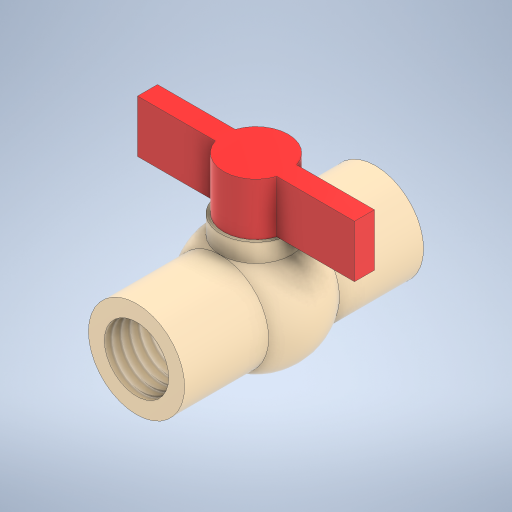
# Autodesk Inventor part: LlaveDesecho
Saved by Autodesk Inventor 2024 (Build 280153000, 153)
## iProperties
Created: 2024-05-01
Part Number: LlaveDesecho
Material: Genérico
Document SubType Name: Modeling
Designer: alexa
Density: 1 g/cm^3
Appearance: Valor por defecto
Author: alexa
Autodesk Inventor part; units mm, degrees
ref_plane "YZ Plane" through (0, 0, 0) normal (1, 0, 0) x (0, 1, 0)
ref_plane "XY Plane" through (0, 0, 0) normal (0, 0, 1) x (1, 0, 0)
sketch "Sketch1" plane through (0, 0, 0) normal (0, 1, 0) x (-1, 0, 0)
  line L0 (0, 0) -> (0, -39)
  line L1 (0, -39) -> (-15.7, -39)
  line L2 (-15.7, 39) -> (0, 39)
  line L3 (0, 39) -> (0, 0)
  arc A0 (-15.7, 11.5655) -> (-15.7, -11.5655) centre (0, 0) ccw
  line L4 (-15.7, -39) -> (-15.7, -11.5655)
  line L5 (-15.7, 11.5655) -> (-15.7, 39)
  dimension "d0" = 39
  dimension "d1" = 15.7
  dimension "d2" = 78
  dimension "d3" = 39
  constraints: 12 end point, 6 perpendicular, 2 point on circle, 1 centre point, 1 coincident, 1 point on line, 1 vertical
  measures "d0" distance of L0.start L0.end
  measures "d1" distance of L0.end L1.end
  measures "d2" distance of L1.end L2.start
  measures "d3" diameter of A0
revolve "Revolution1" add sketch "Sketch1" angle 360 about axis through (0, 0, 0) along (0, 0, -1)
ref_plane "Work Plane1" through (0, 15.7, 25.2827) normal (0, 1, 0) x (-1, 0, 0)
split "Split1" plane through (0, 15.7, 25.2827) removes the side toward (0, 1, 0)
sketch "Sketch2" plane through (0, 15.7, 0) normal (0, 1, 0) x (1, 0, 0)
  circle A0 centre (0, 0) radius 11.5655
  line L0 (15.7, 11.5655) -> (-15.7, 11.5655) projected
  point P0 (0, 11.5655)
  constraints: 1 coincident, 1 horizontal, 1 vertical alignment, 1 other
extrude "Extrusion1" add sketch "Sketch2" along normal blind 6
sketch "Sketch3" plane through (0, 0, 39) normal (0, 0, 1) x (1, 0, 0)
  circle A0 centre (0, 0) radius 10.5
  dimension "d7" = 21
  constraints: 1 centre point, 1 coincident
  measures "d7" diameter of A0
extrude "Extrusion2" cut sketch "Sketch3" against normal blind 78
thread "Thread1" size "M22x3" class "6H" standard "ANSI Metric M Profile" full length
sketch "Sketch4" plane through (0, 21.7, 0) normal (0, 1, 0) x (1, 0, 0)
  line L0 (35.4, -3.25) -> (35.4, 3.25)
  line L1 (-35.4, 3.25) -> (-35.4, -3.25)
  line L2 (35.4, 3.25) -> (10.0369, 3.25)
  line L3 (-10.0369, 3.25) -> (-35.4, 3.25)
  line L4 (-35.4, -3.25) -> (-10.0369, -3.25)
  line L5 (10.0369, -3.25) -> (35.4, -3.25)
  arc A0 (-10.0369, -3.25) -> (10.0369, -3.25) centre (0, 0) ccw
  arc A1 (10.0369, 3.25) -> (-10.0369, 3.25) centre (0, 0) ccw
  dimension "d12" = 70.8
  dimension "d13" = 6.5
  constraints: 12 end point, 5 parallel, 4 point on circle, 2 centre point, 2 horizontal, 2 perpendicular, 1 coincident
  measures "d12" distance of L1.start L0.end
  measures "d13" distance of L0.end L0.start
extrude "Extrusion3" add sketch "Sketch4" along normal blind 17.1
body "Solid1"
